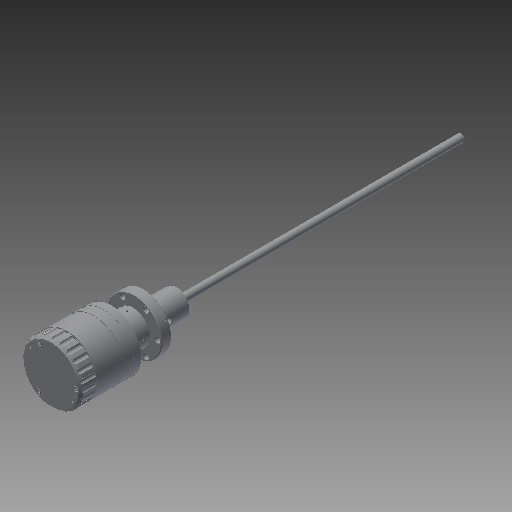
# Autodesk Inventor part: rotary feedthrough (MDC 670024) length extension
Saved by Autodesk Inventor 2018 (Build 220112000, 112)
## iProperties
Created: 2015-02-04
Part Number: rotary feedthrough (MDC 670024) length extension
Material: Generic
Document SubType Name: Modeling
Designer: Pascal
Density: 1 g/cm^3
Appearance: Default
Author: AES
Title: 670024 rev B.STEP
Description: STEP AP203
Creation Date: 2011-08-10
Sending System: SolidWorks 2010
Preprocessor: SwSTEP 2.0
Author: Pascal
Autodesk Inventor part; units mm, degrees
ref_plane "YZ Plane" through (0, 0, 0) normal (1, 0, 0) x (0, 1, 0)
ref_plane "XZ Plane" through (0, 0, 0) normal (0, 1, 0) x (-1, 0, 0)
ref_plane "XY Plane" through (0, 0, 0) normal (0, 0, 1) x (1, 0, 0)
surface "Composite1"
sketch "Sketch1" plane through (0, 0, -260.35) normal (0, 0, -1) x (-1, 0, 0)
  circle A0 centre (0, 0) radius 4.7625
  dimension "d13" = 9.525
  constraints: 1 centre point, 1 coincident
  measures "d13" diameter of A0
extrude "Extrusion1" add sketch "Sketch1" along normal blind 146.05
hole "Hole1" at (0, 0, -406.4) direction (0, 0, 1) diameter 5.3594 depth 12.7 countersink diameter 7.112 countersink angle 57.296 thread size "1/4-28 UNF" class "2B" standard "ANSI Unified Screw Threads"
body "Solid1"
body "Srf1"
